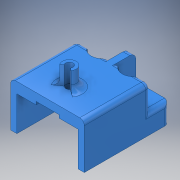
# Autodesk Inventor part: cover_dis
Saved by Autodesk Inventor 2018 (Build 220112000, 112)
## iProperties
Created: 2019-01-15
Part Number: cover_dis
Material: Generic
Document SubType Name: Modeling
Designer: Koki
Density: 1 g/cm^3
Appearance: Cyan
Author: Koki
Autodesk Inventor part; units mm, degrees
ref_plane "YZ Plane" through (0, 0, 0) normal (1, 0, 0) x (0, 1, 0)
ref_plane "XZ Plane" through (0, 0, 0) normal (0, 1, 0) x (-1, 0, 0)
sketch "Sketch1" plane through (0, 0, 0) normal (0, 1, 0) x (-1, 0, 0)
  line L0 (12.05, 13.9095) -> (-12.05, 13.9095)
  line L1 (-12.05, 13.9095) -> (-12.05, -13.9095)
  line L2 (-12.05, -13.9095) -> (12.05, -13.9095)
  line L3 (12.05, -13.9095) -> (12.05, 13.9095)
  point P0 (0, 0)
  dimension "d0" = 24.1
  dimension "d1" = 12.05
  dimension "d2" = 27.819
  dimension "d3" = 13.9095
  constraints: 8 end point, 2 parallel, 1 horizontal, 1 perpendicular
  measures "d0" distance of L0.start L0.end
  measures "d1" distance from line of point (0, 0) L3
  measures "d2" distance of L2.end L0.start
  measures "d3" distance from line of point (0, 0) L2
extrude "Extrusion1" add sketch "Sketch1" against normal blind 13.3
sketch "Sketch2" plane through (0, -13.3, 0) normal (0, -1, 0) x (1, 0, 0)
  line L0 (10.05, 13.9095) -> (-10.05, 13.9095)
  line L1 (-10.05, 13.9095) -> (-10.05, -11.9095)
  line L2 (-10.05, -11.9095) -> (10.05, -11.9095)
  line L3 (10.05, -11.9095) -> (10.05, 13.9095)
  line L4 (12.05, 13.9095) -> (-12.05, 13.9095) projected
  line L5 (12.05, -13.9095) -> (12.05, 13.9095) projected
  line L6 (-12.05, 13.9095) -> (-12.05, -13.9095) projected
  line L7 (-12.05, -13.9095) -> (12.05, -13.9095) projected
  point P0 (0, 0)
  dimension "d6" = 2
  dimension "d7" = 2
  dimension "d8" = 2
  constraints: 8 end point, 2 parallel, 1 horizontal, 1 perpendicular, 1 point on line
  measures "d6" distance between parallel lines of L3 L5
  measures "d7" distance between parallel lines of L6 L1
  measures "d8" distance between parallel lines of L7 L2
extrude "Extrusion2" cut sketch "Sketch2" against normal blind 10.8 contours L3 L2 L1 L0
sketch "Sketch3" plane through (0, 0, 0) normal (0, 1, 0) x (1, 0, 0)
  line L0 (-12.05, 5.7095) -> (12.05, 5.7095)
  line L1 (12.05, 5.7095) -> (12.05, 13.9095)
  line L2 (12.05, 13.9095) -> (-12.05, 13.9095)
  line L3 (-12.05, 13.9095) -> (-12.05, 5.7095)
  point P0 (0, 0)
  dimension "d11" = 8.2
  constraints: 8 end point, 2 coincident, 2 parallel, 1 horizontal, 1 perpendicular
  measures "d11" distance of L2.end L0.start
extrude "Extrusion3" cut sketch "Sketch3" against normal blind 10.3
sketch "Sketch4" plane through (0, -10.3, 0) normal (0, 1, 0) x (1, 0, 0)
  line L0 (-1.1, 5.7095) -> (-12.05, 5.7095)
  line L1 (-12.05, 5.7095) -> (-12.05, 13.9095)
  line L2 (-12.05, 13.9095) -> (-1.1, 13.9095)
  line L3 (-1.1, 13.9095) -> (-1.1, 5.7095)
  point P0 (0, 0)
  dimension "d14" = 10.95
  constraints: 8 end point, 2 coincident, 2 parallel, 1 horizontal, 1 perpendicular
  measures "d14" distance of L1.end L2.end
extrude "Extrusion4" add sketch "Sketch4" along normal blind 2
mirror "Mirror1" about plane through (0, 0, 0) normal (1, 0, 0) of "Extrusion4"
sketch "Sketch6" plane through (0, -13.3, 0) normal (0, -1, 0) x (1, 0, 0)
  line L0 (-12.05, -5.7095) -> (12.05, -5.7095)
  line L1 (12.05, -5.7095) -> (12.05, -13.9095)
  line L2 (12.05, -13.9095) -> (-12.05, -13.9095)
  line L3 (-12.05, -13.9095) -> (-12.05, -5.7095)
  point P0 (0, 0)
  constraints: 8 end point, 3 coincident, 2 parallel, 1 horizontal, 1 perpendicular
extrude "Extrusion6" add sketch "Sketch6" along normal blind 2
sketch "Sketch7" plane through (12.05, 0, -5.7095) normal (0, 0, -1) x (-1, 0, 0)
  line L0 (0, 0) -> (10.95, 0)
  line L1 (10.95, 0) -> (10.95, -8.3)
  line L2 (10.95, -8.3) -> (0, -8.3)
  line L3 (0, -8.3) -> (0, 0)
  point P0 (12.05, 0)
  constraints: 8 end point, 2 coincident, 2 parallel, 1 horizontal, 1 perpendicular
extrude "Extrusion7" add sketch "Sketch7" along normal blind 2
mirror "Mirror3" about plane through (0, 0, 0) normal (1, 0, 0) of "Extrusion7"
sketch "Sketch8" plane through (1.1, -8.3, -13.9095) normal (0, 1, 0) x (1, 0, 0)
  circle A0 centre (4, -4.719) radius 2.25
  line L0 (0, -8.2) -> (8.95, -8.2) projected
  line L1 (8.95, -27.819) -> (8.95, -8.2) projected
  line L2 (10.95, -27.819) -> (10.95, -6.2) projected
  line L3 (8.95, -2) -> (0, -2) projected
  point P0 (-1.1, -13.9095)
  dimension "d24" = 4.5
  dimension "d29" = 6.95
  dimension "d30" = 2.719
  constraints: 1 centre point
  measures "d24" diameter of A0
  measures "d29" distance from line of L2 A0.centre
  measures "d30" distance from line of L3 A0.centre
extrude "Extrusion8" cut sketch "Sketch8" against normal through all
mirror "Mirror4" about plane through (0, 0, 0) normal (1, 0, 0) of "Extrusion8"
sketch "Sketch9" plane through (0, 0, 0) normal (0, 1, 0) x (1, 0, 0)
  circle A0 centre (0, -6.7795) radius 1.15
  line L0 (-12.05, -13.9095) -> (12.05, -13.9095) projected
  circle A1 centre (0, -6.7795) radius 2.25
  point P0 (0, 0)
  dimension "d31" = 7.13
  dimension "d32" = 2.3
  dimension "d33" = 4.5
  constraints: 2 centre point, 1 coincident
  measures "d31" distance from line of A0.centre L0
  measures "d32" diameter of A0
  measures "d33" diameter of A1
extrude "Extrusion9" add sketch "Sketch9" along normal blind 6.1
sketch "Sketch10" plane through (0, 6.1, 6.7795) normal (0, 1, 0) x (1, 0, 0)
  circle A0 centre (0, 0) radius 1.15 projected
  arc A1 (-0.942, -0.6596) -> (0.942, -0.6596) centre (0, 0) ccw
  circle A2 centre (0, 0) radius 2.25 projected
  arc A3 (-1.8431, -1.2905) -> (1.8431, -1.2905) centre (0, 0) ccw
  line L0 (0, 0) -> (-0.8052, 0)
  line L1 (0, 0) -> (0.4727, 0)
  line L2 (0, 0) -> (-0.942, -0.6596)
  line L3 (0, 0) -> (0.942, -0.6596)
  line L4 (-1.8431, -1.2905) -> (-0.942, -0.6596)
  line L5 (0.942, -0.6596) -> (1.8431, -1.2905)
  point P0 (0, 6.7795)
  dimension "d36" = 35
  dimension "d37" = 35
  constraints: 12 end point, 6 point on circle, 2 centre point, 2 coincident, 2 collinear, 1 concentric, 1 horizontal, 1 point on line, 2 other
  measures "d36" angle of L0 L2
  measures "d37" angle of L1 L3
extrude "Extrusion10" cut sketch "Sketch10" against normal up to surface (6.1 mm away) contours A0 L5 A2 L4 picked at (-0.2694, -1.8509)
sketch "Sketch11" plane through (0, 0, 0) normal (0, 1, 0) x (1, 0, 0)
  line L0 (1.1, 5.7095) -> (-1.1, 5.7095) projected
  line L1 (-1.1, 5.7095) -> (-1.1, 7.7095) projected
  line L2 (-1.1, 7.7095) -> (-12.05, 7.7095) projected
  line L3 (-12.05, 7.7095) -> (-12.05, -13.9095) projected
  line L4 (-12.05, -13.9095) -> (12.05, -13.9095) projected
  line L5 (12.05, -13.9095) -> (12.05, 7.7095) projected
  line L6 (1.1, 7.7095) -> (12.05, 7.7095) projected
  line L7 (1.1, 5.7095) -> (1.1, 7.7095) projected
  arc A0 (0.942, -7.4391) -> (-0.942, -7.4391) centre (0, -6.7795) ccw projected
  line L8 (-0.942, -7.4391) -> (-1.8431, -8.07) projected
  arc A1 (1.8431, -8.07) -> (-1.8431, -8.07) centre (0, -6.7795) ccw projected
  line L9 (1.8431, -8.07) -> (0.942, -7.4391) projected
  circle A2 centre (0, -6.7795) radius 1.15
  point P0 (0, 0)
  constraints: 1 centre point, 1 coincident, 1 concentric
extrude "Extrusion11" cut sketch "Sketch11" against normal through all contours A2 A0
fillet "Fillet1" radius 2 1 edges at (0, 0, 4.5295)
fillet "Fillet2" radius 1.5 10 edges at (12.05, 0, 3.1) (-12.05, 0, 3.1) (6.575, 0, -7.7095) (-6.575, 0, -7.7095) (12.05, -4.15, -7.7095) (12.05, -8.3, -10.8095) (12.05, -11.8, -13.9095) (-12.05, -11.8, -13.9095) (-12.05, -8.3, -10.8095) (-12.05, -4.15, -7.7095)
sketch "Sketch12" plane through (0, -8.3, 0) normal (0, 1, 0) x (1, 0, 0)
  arc A0 (-3.4061, 7.7095) -> (-6.7939, 7.7095) centre (-5.1, 9.1905) ccw projected
  arc A1 (6.7939, 7.7095) -> (3.4061, 7.7095) centre (5.1, 9.1905) ccw projected
  circle A2 centre (-5.1, 9.1905) radius 2.25
  circle A3 centre (5.1, 9.1905) radius 2.25
  point P0 (0, 0)
  constraints: 2 centre point, 2 coincident, 2 concentric
extrude "Extrusion12" cut sketch "Sketch12" along normal through all both and the other way through all
sketch "Sketch13" plane through (0, -8.3, 0) normal (0, 1, 0) x (1, 0, 0)
  arc A0 (-3.4061, 7.7095) -> (-6.7939, 7.7095) centre (-5.1, 9.1905) ccw projected
  circle A1 centre (-5.1, 9.1905) radius 3.7
  arc A2 (6.7939, 7.7095) -> (3.4061, 7.7095) centre (5.1, 9.1905) ccw projected
  circle A3 centre (5.1, 9.1905) radius 3.7
  point P0 (0, 0)
  dimension "d46" = 7.4
  dimension "d47" = 7.4
  constraints: 2 centre point, 2 coincident
  measures "d46" diameter of A1
  measures "d47" diameter of A3
extrude "Extrusion13" cut sketch "Sketch13" along normal through all
sketch "Sketch14" plane through (-10.05, -13.3, -5.7095) normal (0, 0, 1) x (1, 0, 0)
  line L0 (-2, 0) -> (22.1, 0)
  line L1 (22.1, 0) -> (22.1, -2)
  line L2 (22.1, -2) -> (-2, -2)
  line L3 (-2, -2) -> (-2, 0)
  point P0 (10.05, 13.3)
  constraints: 8 end point, 2 coincident, 2 parallel, 1 horizontal, 1 perpendicular
extrude "Extrusion14" cut sketch "Sketch14" along normal through all both and the other way through all
sketch "Sketch16" plane through (0, -13.3, 0) normal (0, -1, 0) x (1, 0, 0)
  line L0 (12.05, -12.4095) -> (12.05, 13.9095) projected
  line L1 (12.05, 13.9095) -> (10.05, 13.9095) projected
  line L2 (10.05, 13.9095) -> (10.05, -11.9095) projected
  line L3 (10.05, -11.9095) -> (-10.05, -11.9095) projected
  line L4 (-10.05, -11.9095) -> (-10.05, 13.9095) projected
  line L5 (-10.05, 13.9095) -> (-12.05, 13.9095) projected
  line L6 (-12.05, 13.9095) -> (-12.05, -12.4095) projected
  arc A0 (-12.05, -12.4095) -> (-10.55, -13.9095) centre (-10.55, -12.4095) ccw projected
  line L7 (10.55, -13.9095) -> (-10.55, -13.9095) projected
  arc A1 (10.55, -13.9095) -> (12.05, -12.4095) centre (10.55, -12.4095) ccw projected
  point P0 (0, 0)
extrude "Extrusion16" add sketch "Sketch16" along normal blind 1
sketch "Sketch17" plane through (0, -2.5, 0) normal (0, -1, 0) x (1, 0, 0)
  line L0 (10.05, -3.0905) -> (3.75, -3.0905)
  line L1 (3.75, -3.0905) -> (3.75, 13.9095)
  line L2 (3.75, 13.9095) -> (10.05, 13.9095)
  line L3 (10.05, 13.9095) -> (10.05, -3.0905)
  line L4 (-3.75, -3.0905) -> (-10.05, -3.0905)
  line L5 (-10.05, -3.0905) -> (-10.05, 13.9095)
  line L6 (-10.05, 13.9095) -> (-3.75, 13.9095)
  line L7 (-3.75, 13.9095) -> (-3.75, -3.0905)
  point P0 (0, 0)
  dimension "d57" = 7.5
  dimension "d58" = 6.3
  dimension "d59" = 17
  constraints: 16 end point, 4 parallel, 2 coincident, 2 horizontal, 2 perpendicular, 2 point on line
  measures "d57" distance between parallel lines of L7 L1
  measures "d58" distance of L0.start L0.end
  measures "d59" distance of L0.end L1.end
extrude "Extrusion17" add sketch "Sketch17" along normal blind 1
sketch "Sketch18" plane through (0, -10.3, 0) normal (0, 1, 0) x (1, 0, 0)
  arc A0 (2.9083, 6.2095) -> (7.2917, 6.2095) centre (5.1, 9.1905) ccw projected
  arc A1 (-7.2917, 6.2095) -> (-2.9083, 6.2095) centre (-5.1, 9.1905) ccw projected
  line L0 (-1.1, 13.9095) -> (1.1, 13.9095)
  line L1 (1.1, 13.9095) -> (1.1, 5.7095)
  line L2 (1.1, 5.7095) -> (-1.1, 5.7095)
  line L3 (-1.1, 5.7095) -> (-1.1, 13.9095)
  point P0 (0, 0)
  point P1 (-1.7093, 7.7095)
  constraints: 8 end point, 2 coincident, 2 parallel, 1 horizontal, 1 perpendicular, 1 other
extrude "Extrusion18" add sketch "Sketch18" along normal up to surface (10.3 mm away)
fillet "Fillet3" radius 2 1 edges at (0, 0, -13.9095)
sketch "Sketch19" plane through (0, 6.1, 0) normal (0, 1, 0) x (1, 0, 0)
  arc A0 (0.942, -7.4391) -> (-0.942, -7.4391) centre (0, -6.7795) ccw projected
  circle A1 centre (0, -6.7795) radius 1.225
  point P0 (0, 0)
  dimension "d65" = 2.45
  constraints: 1 centre point, 1 coincident
  measures "d65" diameter of A1
extrude "Extrusion19" cut sketch "Sketch19" against normal up to surface (6.1 mm away)
sketch "Sketch20" plane through (0, 6.1, 0) normal (0, 1, 0) x (1, 0, 0)
  arc A0 (1.0035, -7.4821) -> (-1.0035, -7.4821) centre (0, -6.7795) ccw projected
  line L0 (1.0035, -7.4821) -> (1.8431, -8.07) projected
  arc A1 (1.8431, -8.07) -> (-1.8431, -8.07) centre (0, -6.7795) ccw projected
  line L1 (-1.8431, -8.07) -> (-1.0035, -7.4821) projected
  point P0 (0, 0)
extrude "Extrusion20" [suppressed]
ref_plane "Work Plane1" through (0, 2, 0) normal (0, 1, 0) x (1, 0, 0)
sketch "Sketch22" plane through (0, -14.3, 0) normal (0, -1, 0) x (1, 0, 0)
  line L0 (12.05, -12.4095) -> (12.05, 13.9095) projected
  line L1 (12.05, 13.9095) -> (10.05, 13.9095) projected
  line L2 (10.05, 13.9095) -> (10.05, -11.9095) projected
  line L3 (10.05, -11.9095) -> (-10.05, -11.9095) projected
  line L4 (-10.05, -11.9095) -> (-10.05, 13.9095) projected
  line L5 (-10.05, 13.9095) -> (-12.05, 13.9095) projected
  line L6 (-12.05, 13.9095) -> (-12.05, -12.4095) projected
  arc A0 (-12.05, -12.4095) -> (-10.55, -13.9095) centre (-10.55, -12.4095) ccw projected
  line L7 (-10.55, -13.9095) -> (10.55, -13.9095) projected
  arc A1 (10.55, -13.9095) -> (12.05, -12.4095) centre (10.55, -12.4095) ccw projected
  point P0 (0, 0)
extrude "Extrusion22" add sketch "Sketch22" along normal blind 0.5
equation "\"d1\" = 0.5 * d0"
equation "\"d3\" = 0.5 * d2"
equation "\"d37\" = d36"
body "Solid1"
